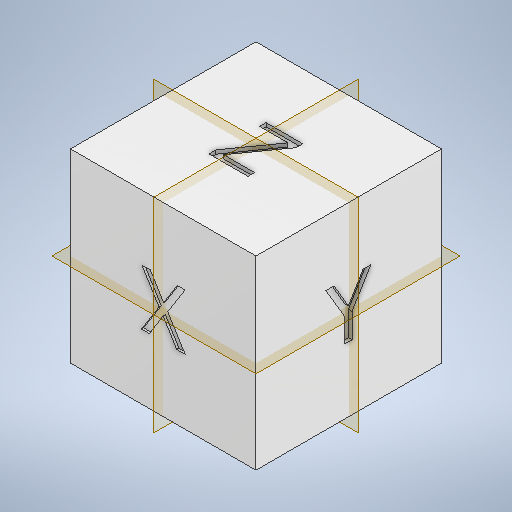
# Autodesk Inventor part: Cubo-0001-001
Saved by Autodesk Inventor 2025.2 (Build 292293000, 293)
## iProperties
Created: 2024-03-21
Part Number: Cubo-0001-001
Material: PCL plástico
Document SubType Name: Modeling
Designer: MiguelBarbosa
Density: 1.626 g/cm^3
Appearance: Suave - Branco
Author: MiguelBarbosa
## iProperties of the stored document _3DPrint.ipt
Created: 2024-03-21
Part Number: _3DPrint
Material: Generic
Document SubType Name: Modeling
Designer: MiguelBarbosa
Density: 1 g/cm^3
Appearance: Default
Author: MiguelBarbosa
Autodesk Inventor part; units mm, degrees
sketch "Sketch1" plane through (0, 0, 0) normal (0, 0, 1) x (1, 0, 0)
  line L0 (-25, -25) -> (25, -25)
  line L1 (25, -25) -> (25, 25)
  line L2 (25, 25) -> (-25, 25)
  line L3 (-25, 25) -> (-25, -25)
  line L4 (-25, -25) -> (25, 25) construction
  line L5 (25, -25) -> (-25, 25) construction
  point P0 (0, 0)
  dimension "d15" = 50
  dimension "d18" = 50
  constraints: 12 end point, 2 midpoint, 2 parallel, 1 horizontal, 1 perpendicular
  measures "d15" distance of L1.end L2.end
  measures "d18" distance of L2.end L0.start
extrude "Extrusion1" add sketch "Sketch1" along normal mid plane 50
sketch "Sketch2" plane through (0, 0, 25) normal (0, 0, 1) x (1, 0, 0)
  line L0 (-5.9866, 7.5) -> (5.9866, 7.5) construction
  line L1 (5.9866, 7.5) -> (5.9866, -7.5) construction
  line L2 (5.9866, -7.5) -> (-5.9866, -7.5) construction
  line L3 (-5.9866, -7.5) -> (-5.9866, 7.5) construction
  line L4 (-5.9866, 7.5) -> (5.9866, -7.5) construction
  line L5 (5.9015, -7.5) -> (3.6163, -7.5)
  line L6 (3.6163, -7.5) -> (-0.0304, -1.5194)
  line L7 (-0.0304, -1.5194) -> (-3.75, -7.5)
  line L8 (-3.75, -7.5) -> (-5.9015, -7.5)
  line L9 (-5.9015, -7.5) -> (-1.1244, 0.0122)
  line L10 (-1.1244, 0.0122) -> (-5.7557, 7.5)
  line L11 (-5.7557, 7.5) -> (-3.4704, 7.5)
  line L12 (-3.4704, 7.5) -> (0.1033, 1.6288)
  line L13 (0.1033, 1.6288) -> (3.75, 7.5)
  line L14 (3.75, 7.5) -> (5.9015, 7.5)
  line L15 (5.9015, 7.5) -> (1.2095, 0.1094)
  line L16 (1.2095, 0.1094) -> (5.9015, -7.5)
  point P0 (0, 0)
  point P1 (0, 0)
  point P2 (0, 0)
  point P3 (0, 0)
  dimension "d3" = 11.9733
  dimension "d4" = 15
  constraints: 3 coincident, 2 end point, 1 horizontal, 1 midpoint, 2 other
  measures "d3" distance of L0.start L0.end
  measures "d4" distance of L2.end L0.start
extrude "Extrusion2" cut sketch "Sketch2" against normal blind 0.6
sketch "Sketch3" plane through (25, -25, 25) normal (1, 0, 0) x (0, 0, -1)
  line L0 (18.9344, 32.5) -> (31.0656, 32.5) construction
  line L1 (31.0656, 32.5) -> (31.0656, 17.5) construction
  line L2 (31.0656, 17.5) -> (18.9344, 17.5) construction
  line L3 (18.9344, 17.5) -> (18.9344, 32.5) construction
  line L4 (31.0656, 32.5) -> (18.9344, 17.5) construction
  line L5 (30.9562, 32.5) -> (25.8874, 24.137)
  line L6 (25.8874, 24.137) -> (25.8874, 17.5)
  line L7 (25.8874, 17.5) -> (23.8938, 17.5)
  line L8 (23.8938, 17.5) -> (23.8938, 23.9303)
  line L9 (23.8938, 23.9303) -> (18.825, 32.5)
  line L10 (18.825, 32.5) -> (21.0373, 32.5)
  line L11 (21.0373, 32.5) -> (24.9028, 25.8995)
  line L12 (24.9028, 25.8995) -> (28.8412, 32.5)
  line L13 (28.8412, 32.5) -> (30.9562, 32.5)
  point P0 (25, 25)
  point P1 (25, 25)
  dimension "d7" = 12.1313
  dimension "d8" = 15
  constraints: 2 end point, 1 coincident, 1 horizontal, 1 midpoint, 2 other
  measures "d7" distance of L0.start L0.end
  measures "d8" distance of L0.end L1.end
extrude "Extrusion3" cut sketch "Sketch3" against normal blind 1
sketch "Sketch4" plane through (-25, 25, 25) normal (0, 1, 0) x (1, 0, 0)
  line L0 (19.2322, 32.5) -> (30.7678, 32.5) construction
  line L1 (30.7678, 32.5) -> (30.7678, 17.5) construction
  line L2 (30.7678, 17.5) -> (19.2322, 17.5) construction
  line L3 (19.2322, 17.5) -> (19.2322, 32.5) construction
  line L4 (30.7678, 32.5) -> (19.2322, 17.5) construction
  line L5 (30.3181, 17.5) -> (19.84, 17.5)
  line L6 (19.84, 17.5) -> (19.84, 19.3598)
  line L7 (19.84, 19.3598) -> (27.8626, 30.7253)
  line L8 (27.8626, 30.7253) -> (20.2046, 30.7253)
  line L9 (20.2046, 30.7253) -> (20.2046, 32.5)
  line L10 (20.2046, 32.5) -> (30.1114, 32.5)
  line L11 (30.1114, 32.5) -> (30.1114, 30.701)
  line L12 (30.1114, 30.701) -> (22.0036, 19.2747)
  line L13 (22.0036, 19.2747) -> (30.3181, 19.2747)
  line L14 (30.3181, 19.2747) -> (30.3181, 17.5)
  point P0 (25, 25)
  point P1 (25, 25)
  dimension "d11" = 11.5357
  dimension "d12" = 15
  constraints: 2 end point, 1 coincident, 1 horizontal, 1 midpoint, 2 other
  measures "d11" distance of L0.start L0.end
  measures "d12" distance of L0.end L1.end
extrude "Extrusion4" cut sketch "Sketch4" against normal blind 1
equation "\"d18\" = d15"
equation "\"d1\" = d15"
body "Solid1"
